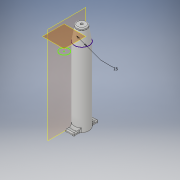
# Autodesk Inventor part: heating
Saved by Autodesk Inventor 2018 (Build 220112000, 112)
## iProperties
Created: 2018-10-08
Part Number: heating
Material: Generic
Document SubType Name: Modeling
Designer: Iek Man Lei
Density: 1 g/cm^3
Appearance: Default
Author: Iek Man Lei
Autodesk Inventor part; units mm, degrees
ref_plane "XZ Plane" through (0, 0, 0) normal (0, 1, 0) x (-1, 0, 0)
ref_plane "XY Plane" through (0, 0, 0) normal (0, 0, 1) x (1, 0, 0)
sketch "Sketch1" plane through (0, 0, 0) normal (0, 1, 0) x (-1, 0, 0)
  circle A0 centre (0, 0) radius 7.5
  circle A1 centre (0, 0) radius 5.5
  dimension "d0" = 15
  dimension "d1" = 11
  constraints: 2 centre point, 2 coincident
  measures "d0" diameter of A0
  measures "d1" diameter of A1
sketch "Sketch2" plane through (0, 0, 0) normal (0, 1, 0) x (-1, 0, 0)
  line L0 (4.5, 12.5) -> (-4.5, 12.5)
  line L1 (-4.5, 12.5) -> (-4.5, -12.5)
  line L2 (-4.5, -12.5) -> (4.5, -12.5)
  line L3 (4.5, -12.5) -> (4.5, 12.5)
  point P0 (0, 0)
  dimension "d2" = 9
  dimension "d3" = 25
  dimension "d4" = 12.5
  dimension "d45" = 4.5
  constraints: 8 end point, 2 parallel, 1 horizontal, 1 perpendicular
  measures "d2" distance of L0.start L0.end
  measures "d3" distance of L0.end L1.end
  measures "d4" distance from line of point (0, 0) L0
  measures "d45" distance from line of point (0, 0) L3
extrude "Extrusion1" add sketch "Sketch2" along normal blind 3
extrude "Extrusion2" add sketch "Sketch1" along normal blind 76
sketch "Sketch3" plane through (0, 0, 0) normal (0, -1, 0) x (1, 0, 0)
  circle A0 centre (0, 0) radius 5.5
  dimension "d9" = 11
  constraints: 1 centre point, 1 coincident
  measures "d9" diameter of A0
extrude "Extrusion3" cut sketch "Sketch3" against normal blind 76
sketch "Sketch9" plane through (0, 76, 0) normal (0, 1, 0) x (1, 0, 0)
  circle A0 centre (0, -17.8864) radius 4.6199
  point P0 (0, 0)
  constraints: 1 centre point
ref_plane "Work Plane2" through (0, 89, 17.8864) normal (0, 1, 0) x (1, 0, 0)
sketch "Sketch10" plane through (0, 89, 17.8864) normal (0, 1, 0) x (1, 0, 0)
  circle A0 centre (0, 17.8864) radius 3.25
  dimension "d18" = 6.5
  constraints: 1 centre point, 1 coincident
  measures "d18" diameter of A0
sketch "Sketch11" plane through (0, 76, 0) normal (0, 1, 0) x (1, 0, 0)
  circle A0 centre (0, 0) radius 5.5
  constraints: 1 centre point, 1 coincident
sketch "Sketch12" plane through (0, 76, 0) normal (0, 1, 0) x (1, 0, 0)
  circle A0 centre (0, 0) radius 7.5
  dimension "d46" = 15
  constraints: 1 centre point, 1 coincident
  measures "d46" diameter of A0
ref_plane "Work Plane3" through (0, 89, 17.8864) normal (0, 1, 0) x (1, 0, 0)
sketch "Sketch13" plane through (0, 89, 17.8864) normal (0, 1, 0) x (1, 0, 0)
  circle A0 centre (0, 17.8864) radius 5.25
  dimension "d23" = 10.5
  constraints: 1 centre point, 1 coincident
  measures "d23" diameter of A0
loft "Loft2" add profiles "Sketch13" section 1 edges at (7.5, 76, 0)
loft "Loft3" cut profiles "Sketch10" section 1 edges at (0, 76, -5.5) (0, 76, 5.5)
fillet "Fillet1" radius 2 6 edges at (0, 3, 7.5) (0, 3, -7.5) (4.5, 1.5, 6) (4.5, 1.5, -6) (-4.5, 1.5, 6) (-4.5, 1.5, -6)
ref_plane "Work Plane1" through (-10, 0, 0) normal (1, 0, 0) x (0, 1, 0)
sketch "Sketch14" plane through (-10, 0, 0) normal (1, 0, 0) x (0, 1, 0)
  circle A0 centre (64, 0) radius 2.5
  line L0 (76, -7.5) -> (76, 7.5) projected
  point P0 (0, 0)
  dimension "d36" = 12
  dimension "d37" = 5
  constraints: 1 centre point
  measures "d36" distance from line of A0.centre L0
  measures "d37" diameter of A0
extrude "Extrusion6" cut sketch "Sketch14" along normal blind 13
fillet "Fillet2" radius 1 31 edges at (4.5, 3.11, -7.6158) (4.6871, 4.1714, -6.0835) (4.5, 3, -10.4333) (4.5, 3.11, 7.6158) (4.6871, 4.1714, 6.0835) (4.5, 3, 10.4333) (4.6647, 0, 6.1335) (7.5, 0, 0) (4.6647, 0, -6.1335) (4.5, 0, -9.7141) (4.5, 0, 9.7141) (4.5, 1.5, 12.5) (4.5, 1.5, -12.5) (0, 0, 12.5) (0, 3, 12.5) (-4.6647, 0, 6.1335) (-6.8825, 0, -2.9802) (-6.8825, 0, 2.9802) (-4.6647, 0, -6.1335) (-4.5, 0, -9.7141) (-4.5, 0, 9.7141) (0, 0, -12.5) (-4.5, 3.11, 7.6158) (-4.6871, 4.1714, 6.0835) (-4.5, 3, 10.4333) (-4.6871, 4.1714, -6.0835) (-4.5, 3, -10.4333) (-4.5, 3.11, -7.6158) (-4.5, 1.5, -12.5) (-4.5, 1.5, 12.5) (0, 3, -12.5)
sketch "Sketch15" plane through (0, 89, 0) normal (0, 1, 0) x (1, 0, 0)
  circle A0 centre (0, 0) radius 5.25
  dimension "d47" = 10.5
  constraints: 1 centre point, 1 coincident
  measures "d47" diameter of A0
extrude "Extrusion7" add sketch "Sketch15" along normal blind 2
sketch "Sketch16" plane through (0, 91, 0) normal (0, 1, 0) x (1, 0, 0)
  circle A0 centre (0, 0) radius 1.25
  dimension "d41" = 2.5
  constraints: 1 centre point, 1 coincident
  measures "d41" diameter of A0
extrude "Extrusion8" cut sketch "Sketch16" against normal blind 2
fillet "Fillet3" radius 1 3 edges at (0, 89, 5.25) (0, 89, -5.25) (-5.25, 91, 0)
body "Solid1"
